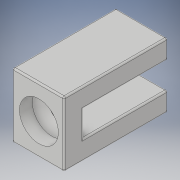
# Autodesk Inventor part: TensionerAxleHolder
Saved by Autodesk Inventor 2017 (Build 210142000, 142)
## iProperties
Created: 2017-07-29
Part Number: TensionerAxleHolder
Material: Generic
Document SubType Name: Modeling
Designer: User
Density: 1 g/cm^3
Appearance: Default
Author: User
Autodesk Inventor part; units mm, degrees
ref_plane "YZ Plane" through (0, 0, 0) normal (1, 0, 0) x (0, 1, 0)
ref_plane "XZ Plane" through (0, 0, 0) normal (0, 1, 0) x (-1, 0, 0)
ref_plane "XY Plane" through (0, 0, 0) normal (0, 0, 1) x (1, 0, 0)
sketch "Sketch1" plane through (0, 0, 0) normal (1, 0, 0) x (0, 1, 0)
  line L0 (0, 0) -> (15.875, 0)
  line L1 (15.875, 0) -> (15.875, -25.4)
  line L2 (0, -25.4) -> (0, 0)
  line L3 (4.7625, -25.4) -> (5.9323, -25.4)
  line L4 (4.7625, -25.4) -> (4.7625, -4.7625)
  line L5 (4.7625, -4.7625) -> (11.1125, -4.7625)
  line L6 (11.1125, -4.7625) -> (11.1125, -25.4)
  line L7 (15.875, -25.4) -> (11.1125, -25.4)
  line L8 (4.7625, -25.4) -> (0, -25.4)
  dimension "d1" = 25.4
  dimension "d4" = 6.35
  dimension "d6" = 4.7625
  dimension "d15" = 25.4
  dimension "d22" = 4.7625
  dimension "d24" = 4.7625
  constraints: 18 end point, 4 parallel, 2 horizontal, 1 perpendicular
  measures "d1" distance of L0.end L1.end
  measures "d4" distance of L4.end L5.end
  measures "d6" distance between parallel lines of L2 L4
  measures "d15" distance of L2.start L0.start
  measures "d22" distance between parallel lines of L1 L6
  measures "d24" distance between parallel lines of L0 L5
extrude "Extrusion1" add sketch "Sketch1" along normal blind 12.7
fillet "Fillet2" radius 0.381 22 edges at (12.7, 15.875, -12.7) (12.7, 11.1125, -15.0813) (0, 15.875, -12.7) (12.7, 7.9375, 0) (12.7, 7.9375, -4.7625) (12.7, 4.7625, -15.0812) (12.7, 0, -12.7) (12.7, 13.4938, -25.4) (12.7, 2.3813, -25.4) (6.35, 15.875, 0) (0, 7.9375, 0) (6.35, 0, 0) (6.35, 15.875, -25.4) (6.35, 4.7625, -25.4) (0, 11.1125, -15.0813) (0, 7.9375, -4.7625) (0, 4.7625, -15.0812) (6.35, 11.1125, -25.4) (0, 13.4938, -25.4) (0, 2.3813, -25.4) (0, 0, -12.7) (6.35, 0, -25.4)
sketch "Sketch6" plane through (0.381, 0.381, 0) normal (0, 0, 1) x (1, 0, 0)
  line L0 (0, 0) -> (0, 15.113) projected
  line L1 (11.938, 0) -> (0, 0) projected
  line L2 (11.938, 15.113) -> (11.938, 0) projected
  line L3 (0, 15.113) -> (11.938, 15.113) projected
  point P0 (-0.381, -0.381)
  point P1 (6.1556, 7.3722)
hole "Hole1" at (6.5366, 7.7532, 0) direction (0, 0, -1) diameter 3.81 end through all
sketch "Sketch7" plane through (0.381, 0.381, 0) normal (0, 0, 1) x (1, 0, 0)
  circle A0 centre (6.1556, 7.3722) radius 1.905 projected
  line L0 (0, 0) -> (0, 15.113) projected
  line L1 (11.938, 0) -> (0, 0) projected
  line L2 (11.938, 15.113) -> (11.938, 0) projected
  line L3 (0, 15.113) -> (11.938, 15.113) projected
  point P0 (-0.381, -0.381)
hole "Hole2" at (6.5366, 7.7532, 0) direction (0, 0, -1) diameter 9.525 depth 3.175 tip angle 118
equation "\"d15\" = d1"
body "Solid1"
